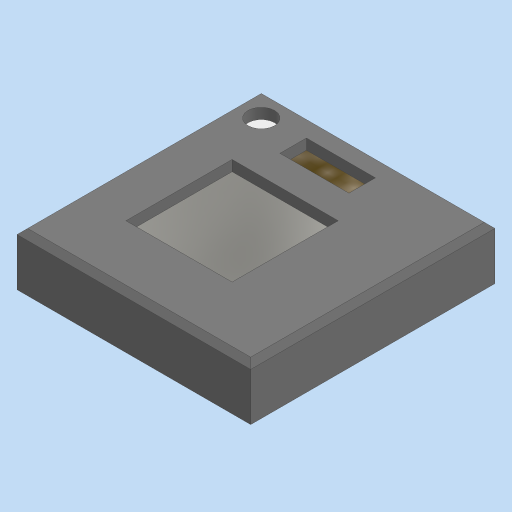
# Autodesk Inventor part: Optical_sensor
Saved by Autodesk Inventor 2024 (Build 280153000, 153)
## iProperties
Created: 2025-02-15
Part Number: Optical_sensor
Material: Generic
Document SubType Name: Modeling
Designer: XxPan
Density: 1 g/cm^3
Appearance: Default
Author: XxPan
Autodesk Inventor part; units mm, degrees
ref_plane "YZ Plane" through (0, 0, 0) normal (1, 0, 0) x (0, 1, 0)
ref_plane "XZ Plane" through (0, 0, 0) normal (0, 1, 0) x (-1, 0, 0)
sketch "Sketch1" plane through (0, 0, 0) normal (0, 1, 0) x (-1, 0, 0)
  line L0 (1.93, 2.3) -> (-2.47, 2.3)
  line L1 (-2.47, 2.3) -> (-2.47, -2.3)
  line L2 (-2.47, -2.3) -> (1.93, -2.3)
  line L3 (1.93, -2.3) -> (1.93, 2.3)
  line L4 (0, -3.22) -> (0, 3.22) construction
  line L5 (2.81, 0) -> (-3.35, 0) construction
  point P0 (0, 0)
  point P1 (-0.27, 2.3)
  point P2 (1.93, 0)
  dimension "d0" = 4.4
  dimension "d1" = 4.6
  dimension "d2" = 0.27
  constraints: 8 end point, 2 midpoint, 2 parallel, 1 horizontal, 1 perpendicular, 1 point on line
  measures "d0" distance of L2.end L1.end
  measures "d1" distance of L1.end L0.end
  measures "d2" distance from line of L4 point (-0.27, 2.3)
extrude "Extrusion1" add sketch "Sketch1" along normal blind 1
sketch "Sketch2" plane through (0, 1, 0) normal (0, 1, 0) x (1, 0, 0)
  line L0 (-1.03, -1.15) -> (0.97, -1.15)
  line L1 (0.97, -1.15) -> (0.97, 0.85)
  line L2 (0.97, 0.85) -> (-1.03, 0.85)
  line L3 (-1.03, 0.85) -> (-1.03, -1.15)
  line L4 (-1.93, 2.3) -> (-1.93, -2.3) projected
  line L5 (-1.93, -2.3) -> (2.47, -2.3) projected
  line L6 (-0.68, 1.4) -> (0.62, 1.4)
  line L7 (0.62, 1.4) -> (0.62, 1.9)
  line L8 (0.62, 1.9) -> (-0.68, 1.9)
  line L9 (-0.68, 1.9) -> (-0.68, 1.4)
  line L10 (2.47, 2.3) -> (-1.93, 2.3) projected
  circle A0 centre (-1.43, 1.8) radius 0.25
  point P0 (0, 0)
  point P1 (-0.03, 0.85)
  point P2 (-0.03, 1.4)
  dimension "d5" = 2
  dimension "d6" = 2
  dimension "d7" = 0.9
  dimension "d8" = 1.15
  dimension "d9" = 0.5
  dimension "d10" = 1.3
  dimension "d11" = 0.4
  dimension "d12" = 0.5
  dimension "d13" = 0.5
  dimension "d14" = 0.5
  constraints: 16 end point, 4 parallel, 2 horizontal, 2 midpoint, 2 perpendicular, 1 centre point, 1 vertical alignment
  measures "d5" distance of L2.end L1.end
  measures "d6" distance of L1.end L0.end
  measures "d7" distance between parallel lines of L3 L4
  measures "d8" distance between parallel lines of L5 L0
  measures "d9" distance of L8.end L6.start
  measures "d10" distance of L6.start L6.end
  measures "d11" distance between parallel lines of L10 L8
  measures "d12" diameter of A0
  measures "d13" distance from line of L4 A0.centre
  measures "d14" distance from line of L10 A0.centre
extrude "Extrusion2" cut sketch "Sketch2" against normal blind 0.2
chamfer "Chamfer1" distance 0.1 angle 45 4 edges at (-1.93, 1, 0) (0.27, 1, -2.3) (2.47, 1, 0) (0.27, 1, 2.3)
ref_plane "Work Plane2" through (0.62, 1, -1.125) normal (0, 0, -1) x (-1, 0, 0)
body "Solid1"
